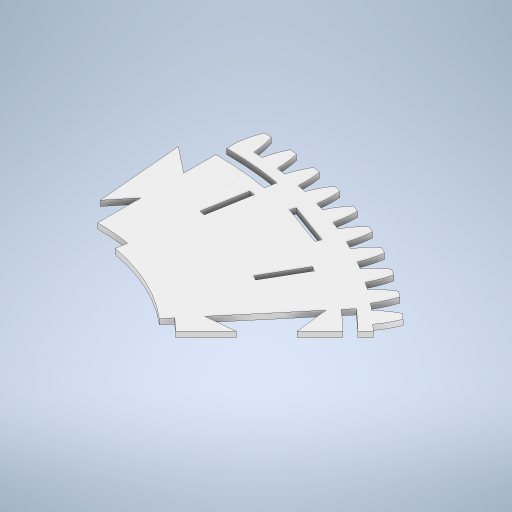
# Autodesk Inventor part: Base Plate Bottom v3
Saved by Autodesk Inventor 2023 (Build 270158000, 158)
## iProperties
Created: 2023-02-13
Part Number: Base Plate Bottom v3
Material: LCP Plastic
Document SubType Name: Sheet Metal
Designer: cheng
Density: 1.626 g/cm^3
Appearance: Smooth - White
Sheet Metal Rule: Default
Author: cheng
Autodesk Inventor part; units mm, degrees
ref_plane "YZ Plane" through (0, 0, 0) normal (1, 0, 0) x (0, 1, 0)
ref_plane "XZ Plane" through (0, 0, 0) normal (0, 1, 0) x (-1, 0, 0)
ref_plane "XY Plane" through (0, 0, 0) normal (0, 0, 1) x (1, 0, 0)
sketch "Sketch2" plane through (0, 0, 0) normal (0, 1, 0) x (-1, 0, 0)
  circle A0 centre (0, 0) radius 325
  circle A1 centre (0, 0) radius 165
  line L0 (0, 0) -> (0, -325)
  line L1 (0, 0) -> (-229.8097, -229.8097)
  line L2 (0, 0) -> (28.3256, -323.7633)
  line L3 (0, 0) -> (-208.906, -248.9644)
  circle A2 centre (0, 0) radius 275 construction
  circle A3 centre (0, 0) radius 195
  circle A4 centre (0, 0) radius 215
  circle A5 centre (0, 0) radius 255 construction
  line L4 (16.9954, -194.258) -> (0, -215)
  line L5 (23.9678, -273.9535) -> (0, -255)
  line L6 (-125.3436, -149.3787) -> (-152.028, -152.028)
  line L7 (-176.7666, -210.6622) -> (-180.3122, -180.3122)
  line L8 (0, 0) -> (-111.1565, -305.4001) construction
  circle A6 centre (0, 0) radius 235 construction
  circle A7 centre (0, 0) radius 275 construction
  line L9 (0, 0) -> (-17.0092, -324.5546) construction
  line L10 (0, 0) -> (-8.5075, -324.8886) construction
  circle A8 centre (0, 0) radius 305
  arc A9 (-5.1732, -324.9588) -> (0, -305) centre (-79.3819, -295.0744) ccw
  arc A10 (-15.9625, -304.582) -> (-11.8409, -324.7842) centre (63.8301, -298.8246) ccw
  arc A11 (20.3387, -324.363) -> (23.93, -304.0598) centre (-55.9859, -300.393) ccw
  arc A12 (7.984, -304.8955) -> (13.6779, -324.712) centre (87.0788, -292.8953) ccw
  arc A13 (45.7252, -321.7673) -> (47.7125, -301.2449) centre (-32.2447, -303.8596) ccw
  arc A14 (31.8812, -303.3292) -> (39.1123, -322.6379) centre (109.7907, -285.1603) ccw
  arc A15 (70.8298, -317.1879) -> (71.2008, -296.5728) centre (-8.3048, -305.4528) ccw
  arc A16 (55.5818, -299.8927) -> (64.3057, -318.5746) centre (131.8257, -275.6672) ccw
  arc A17 (95.4978, -310.6528) -> (94.2502, -290.0722) centre (15.6864, -305.1628) ccw
  arc A18 (78.9398, -294.6074) -> (89.1025, -312.5472) centre (153.0479, -264.4745) ccw
  arc A19 (119.5769, -302.2025) -> (116.7184, -281.7833) centre (39.5808, -302.9913) ccw
  arc A20 (101.8111, -287.5057) -> (113.35, -304.5928) centre (173.3265, -251.6512) ccw
  arc A21 (142.9188, -291.889) -> (138.4671, -271.757) centre (63.2312, -298.9518) ccw
  arc A22 (124.0547, -278.6314) -> (136.8987, -294.7605) centre (192.5365, -237.2764) ccw
  arc A23 (165.3796, -279.776) -> (159.3621, -260.0553) centre (86.4918, -293.0692) ccw
  arc A24 (145.5334, -268.0392) -> (159.6033, -283.1109) centre (210.5595, -221.4387) ccw
  arc A25 (186.8208, -265.938) -> (179.2745, -246.7502) centre (109.2191, -285.3797) ccw
  arc A26 (166.1149, -255.7945) -> (181.3239, -269.7159) centre (227.2843, -204.2358) ccw
  arc A27 (207.1101, -250.4604) -> (198.0817, -231.9238) centre (131.273, -275.9308) ccw
  arc A28 (185.6722, -241.9728) -> (201.9266, -254.6579) centre (242.6078, -185.7736) ccw
  arc A29 (226.1226, -233.4386) -> (215.6676, -215.6676) centre (152.5177, -264.7806) ccw
  arc A30 (204.0848, -226.6592) -> (221.2844, -238.0299) centre (256.4356, -166.1662) ccw
  arc A31 (243.7409, -214.9776) -> (231.9238, -198.0817) centre (172.8219, -251.998) ccw
  arc A32 (221.2392, -209.9481) -> (239.2778, -219.9344) centre (268.6823, -145.5342) ccw
  arc A33 (259.8565, -195.1912) -> (246.7502, -179.2745) centre (192.0607, -237.6617) ccw
  arc A34 (237.0295, -191.9427) -> (255.7961, -200.4829) centre (279.2725, -124.005) ccw
  arc A35 (274.3699, -174.2014) -> (260.0553, -159.3621) centre (210.1154, -221.8601) ccw
  arc A36 (251.3585, -172.7539) -> (270.7372, -179.7953) centre (288.1409, -101.7113) ccw
  arc A37 (287.1918, -152.1376) -> (271.757, -138.4671) centre (226.8746, -204.6908) ccw
  arc A38 (264.1377, -152.5) -> (284.0092, -157.9993) centre (295.2329, -78.7905) ccw
  arc A39 (298.2431, -129.1358) -> (281.7833, -116.7184) centre (242.2351, -186.2594) ccw
  arc A40 (275.2885, -131.3059) -> (295.5302, -135.2291) centre (300.5046, -55.3839) ccw
  arc A41 (307.4556, -105.3378) -> (290.0722, -94.2502) centre (256.1021, -166.6797) ccw
  arc A42 (284.742, -109.3022) -> (305.2291, -111.6252) centre (303.9236, -31.6358) ccw
  arc A43 (314.7725, -80.8904) -> (296.5728, -71.2008) centre (268.3902, -146.0723) ccw
  arc A44 (292.44, -86.6247) -> (313.0462, -87.3331) centre (305.4688, -7.6927) ccw
  arc A45 (320.1488, -55.9443) -> (301.2449, -47.7125) centre (279.0235, -124.5644) ccw
  arc A46 (298.335, -63.4131) -> (318.9333, -62.5025) centre (305.1308, 16.2978) ccw
  arc A47 (323.5512, -30.6533) -> (304.0598, -23.93) centre (287.9366, -102.2884) ccw
  arc A48 (302.3907, -39.8105) -> (322.854, -37.2867) centre (302.9114, 40.1878) ccw
  arc A49 (324.9588, -5.1732) -> (305, 0) centre (295.0744, -79.3819) ccw
  arc A50 (304.582, -15.9625) -> (324.7842, -11.8409) centre (298.8246, 63.8301) ccw
  arc A51 (324.363, 20.3387) -> (304.0598, 23.93) centre (300.393, -55.9859) ccw
  arc A52 (304.8955, 7.984) -> (324.712, 13.6779) centre (292.8953, 87.0788) ccw
  arc A53 (321.7673, 45.7252) -> (301.2449, 47.7125) centre (303.8596, -32.2447) ccw
  arc A54 (303.3292, 31.8812) -> (322.6379, 39.1123) centre (285.1603, 109.7907) ccw
  arc A55 (317.1879, 70.8298) -> (296.5728, 71.2008) centre (305.4528, -8.3048) ccw
  arc A56 (299.8927, 55.5818) -> (318.5746, 64.3057) centre (275.6672, 131.8257) ccw
  arc A57 (310.6528, 95.4978) -> (290.0722, 94.2502) centre (305.1628, 15.6864) ccw
  arc A58 (294.6074, 78.9398) -> (312.5472, 89.1025) centre (264.4745, 153.0479) ccw
  arc A59 (302.2025, 119.5769) -> (281.7833, 116.7184) centre (302.9913, 39.5808) ccw
  arc A60 (287.5057, 101.8111) -> (304.5928, 113.35) centre (251.6512, 173.3265) ccw
  arc A61 (291.889, 142.9188) -> (271.757, 138.4671) centre (298.9518, 63.2312) ccw
  arc A62 (278.6314, 124.0547) -> (294.7605, 136.8987) centre (237.2764, 192.5365) ccw
  arc A63 (279.776, 165.3796) -> (260.0553, 159.3621) centre (293.0692, 86.4918) ccw
  arc A64 (268.0392, 145.5334) -> (283.1109, 159.6033) centre (221.4387, 210.5595) ccw
  arc A65 (265.938, 186.8208) -> (246.7502, 179.2745) centre (285.3797, 109.2191) ccw
  arc A66 (255.7945, 166.1149) -> (269.7159, 181.3239) centre (204.2358, 227.2843) ccw
  arc A67 (250.4604, 207.1101) -> (231.9238, 198.0817) centre (275.9308, 131.273) ccw
  arc A68 (241.9728, 185.6722) -> (254.6579, 201.9266) centre (185.7736, 242.6078) ccw
  arc A69 (233.4386, 226.1226) -> (215.6676, 215.6676) centre (264.7806, 152.5177) ccw
  arc A70 (226.6592, 204.0848) -> (238.0299, 221.2844) centre (166.1662, 256.4356) ccw
  arc A71 (214.9776, 243.7409) -> (198.0817, 231.9238) centre (251.998, 172.8219) ccw
  arc A72 (209.9481, 221.2392) -> (219.9344, 239.2778) centre (145.5342, 268.6823) ccw
  arc A73 (195.1912, 259.8565) -> (179.2745, 246.7502) centre (237.6617, 192.0607) ccw
  arc A74 (191.9427, 237.0295) -> (200.4829, 255.7961) centre (124.005, 279.2725) ccw
  arc A75 (174.2014, 274.3699) -> (159.3621, 260.0553) centre (221.8601, 210.1154) ccw
  arc A76 (172.7539, 251.3585) -> (179.7953, 270.7372) centre (101.7113, 288.1409) ccw
  arc A77 (152.1376, 287.1918) -> (138.4671, 271.757) centre (204.6908, 226.8746) ccw
  arc A78 (152.5, 264.1377) -> (157.9993, 284.0092) centre (78.7905, 295.2329) ccw
  arc A79 (129.1358, 298.2431) -> (116.7184, 281.7833) centre (186.2594, 242.2351) ccw
  arc A80 (131.3059, 275.2885) -> (135.2291, 295.5302) centre (55.3839, 300.5046) ccw
  arc A81 (105.3378, 307.4556) -> (94.2502, 290.0722) centre (166.6797, 256.1021) ccw
  arc A82 (109.3022, 284.742) -> (111.6252, 305.2291) centre (31.6358, 303.9236) ccw
  arc A83 (80.8904, 314.7725) -> (71.2008, 296.5728) centre (146.0723, 268.3902) ccw
  arc A84 (86.6247, 292.44) -> (87.3331, 313.0462) centre (7.6927, 305.4688) ccw
  arc A85 (55.9443, 320.1488) -> (47.7125, 301.2449) centre (124.5644, 279.0235) ccw
  arc A86 (63.4131, 298.335) -> (62.5025, 318.9333) centre (-16.2978, 305.1308) ccw
  arc A87 (30.6533, 323.5512) -> (23.93, 304.0598) centre (102.2884, 287.9366) ccw
  arc A88 (39.8105, 302.3907) -> (37.2867, 322.854) centre (-40.1878, 302.9114) ccw
  circle A89 centre (0, 0) radius 295
  circle A90 centre (0, 0) radius 285
  line L11 (0, 0) -> (-52.9627, -300.3664)
  line L12 (-80.392, -279.3513) -> (-117.9797, -265.6705)
  line L13 (-117.9797, -265.6705) -> (-116.2696, -260.972)
  line L14 (-116.2696, -260.972) -> (-78.6819, -274.6528)
  line L15 (-78.6819, -274.6528) -> (-80.392, -279.3513)
  line L16 (-80.392, -279.3513) -> (-116.2696, -260.972) construction
  line L17 (-117.9797, -265.6705) -> (-78.6819, -274.6528) construction
  line L18 (-98.3308, -270.1616) -> (-99.1858, -272.5109)
  circle A91 centre (0, 0) radius 175
  line L19 (-135.3349, -239.407) -> (-139.6651, -236.907)
  line L20 (-139.6651, -236.907) -> (-119.6651, -202.266)
  line L21 (-119.6651, -202.266) -> (-115.3349, -204.766)
  line L22 (-115.3349, -204.766) -> (-135.3349, -239.407)
  line L23 (-135.3349, -239.407) -> (-119.6651, -202.266) construction
  line L24 (-139.6651, -236.907) -> (-115.3349, -204.766) construction
  line L25 (-137.5, -238.157) -> (-117.5, -203.516) construction
  line L26 (-129.6651, -219.5865) -> (-125.3349, -222.0865) construction
  line L27 (-50.2153, -270.388) -> (-45.2912, -271.2563)
  line L28 (-45.2912, -271.2563) -> (-38.3453, -231.8639)
  line L29 (-38.3453, -231.8639) -> (-43.2693, -230.9957)
  line L30 (-43.2693, -230.9957) -> (-50.2153, -270.388)
  line L31 (-50.2153, -270.388) -> (-38.3453, -231.8639) construction
  line L32 (-45.2912, -271.2563) -> (-43.2693, -230.9957) construction
  line L33 (-47.7532, -270.8221) -> (-40.8073, -231.4298) construction
  arc A92 (5.1732, 324.9588) -> (0, 305) centre (79.3819, 295.0744) ccw
  arc A93 (15.9625, 304.582) -> (11.8409, 324.7842) centre (-63.8301, 298.8246) ccw
  arc A94 (-20.3387, 324.363) -> (-23.93, 304.0598) centre (55.9859, 300.393) ccw
  arc A95 (-7.984, 304.8955) -> (-13.6779, 324.712) centre (-87.0788, 292.8953) ccw
  arc A96 (-45.7252, 321.7673) -> (-47.7125, 301.2449) centre (32.2447, 303.8596) ccw
  arc A97 (-31.8812, 303.3292) -> (-39.1123, 322.6379) centre (-109.7907, 285.1603) ccw
  arc A98 (-70.8298, 317.1879) -> (-71.2008, 296.5728) centre (8.3048, 305.4528) ccw
  arc A99 (-55.5818, 299.8927) -> (-64.3057, 318.5746) centre (-131.8257, 275.6672) ccw
  arc A100 (-95.4978, 310.6528) -> (-94.2502, 290.0722) centre (-15.6864, 305.1628) ccw
  arc A101 (-78.9398, 294.6074) -> (-89.1025, 312.5472) centre (-153.0479, 264.4745) ccw
  arc A102 (-119.5769, 302.2025) -> (-116.7184, 281.7833) centre (-39.5808, 302.9913) ccw
  arc A103 (-101.8111, 287.5057) -> (-113.35, 304.5928) centre (-173.3265, 251.6512) ccw
  arc A104 (-142.9188, 291.889) -> (-138.4671, 271.757) centre (-63.2312, 298.9518) ccw
  arc A105 (-124.0547, 278.6314) -> (-136.8987, 294.7605) centre (-192.5365, 237.2764) ccw
  arc A106 (-165.3796, 279.776) -> (-159.3621, 260.0553) centre (-86.4918, 293.0692) ccw
  arc A107 (-145.5334, 268.0392) -> (-159.6033, 283.1109) centre (-210.5595, 221.4387) ccw
  arc A108 (-186.8208, 265.938) -> (-179.2745, 246.7502) centre (-109.2191, 285.3797) ccw
  arc A109 (-166.1149, 255.7945) -> (-181.3239, 269.7159) centre (-227.2843, 204.2358) ccw
  arc A110 (-207.1101, 250.4604) -> (-198.0817, 231.9238) centre (-131.273, 275.9308) ccw
  arc A111 (-185.6722, 241.9728) -> (-201.9266, 254.6579) centre (-242.6078, 185.7736) ccw
  arc A112 (-226.1226, 233.4386) -> (-215.6676, 215.6676) centre (-152.5177, 264.7806) ccw
  arc A113 (-204.0848, 226.6592) -> (-221.2844, 238.0299) centre (-256.4356, 166.1662) ccw
  arc A114 (-243.7409, 214.9776) -> (-231.9238, 198.0817) centre (-172.8219, 251.998) ccw
  arc A115 (-221.2392, 209.9481) -> (-239.2778, 219.9344) centre (-268.6823, 145.5342) ccw
  arc A116 (-259.8565, 195.1912) -> (-246.7502, 179.2745) centre (-192.0607, 237.6617) ccw
  arc A117 (-237.0295, 191.9427) -> (-255.7961, 200.4829) centre (-279.2725, 124.005) ccw
  arc A118 (-274.3699, 174.2014) -> (-260.0553, 159.3621) centre (-210.1154, 221.8601) ccw
  arc A119 (-251.3585, 172.7539) -> (-270.7372, 179.7953) centre (-288.1409, 101.7113) ccw
  arc A120 (-287.1918, 152.1376) -> (-271.757, 138.4671) centre (-226.8746, 204.6908) ccw
  arc A121 (-264.1377, 152.5) -> (-284.0092, 157.9993) centre (-295.2329, 78.7905) ccw
  arc A122 (-298.2431, 129.1358) -> (-281.7833, 116.7184) centre (-242.2351, 186.2594) ccw
  arc A123 (-275.2885, 131.3059) -> (-295.5302, 135.2291) centre (-300.5046, 55.3839) ccw
  arc A124 (-307.4556, 105.3378) -> (-290.0722, 94.2502) centre (-256.1021, 166.6797) ccw
  arc A125 (-284.742, 109.3022) -> (-305.2291, 111.6252) centre (-303.9236, 31.6358) ccw
  arc A126 (-314.7725, 80.8904) -> (-296.5728, 71.2008) centre (-268.3902, 146.0723) ccw
  arc A127 (-292.44, 86.6247) -> (-313.0462, 87.3331) centre (-305.4688, 7.6927) ccw
  arc A128 (-320.1488, 55.9443) -> (-301.2449, 47.7125) centre (-279.0235, 124.5644) ccw
  arc A129 (-298.335, 63.4131) -> (-318.9333, 62.5025) centre (-305.1308, -16.2978) ccw
  arc A130 (-323.5512, 30.6533) -> (-304.0598, 23.93) centre (-287.9366, 102.2884) ccw
  arc A131 (-302.3907, 39.8105) -> (-322.854, 37.2867) centre (-302.9114, -40.1878) ccw
  arc A132 (-324.9588, 5.1732) -> (-305, 0) centre (-295.0744, 79.3819) ccw
  arc A133 (-304.582, 15.9625) -> (-324.7842, 11.8409) centre (-298.8246, -63.8301) ccw
  arc A134 (-324.363, -20.3387) -> (-304.0598, -23.93) centre (-300.393, 55.9859) ccw
  arc A135 (-304.8955, -7.984) -> (-324.712, -13.6779) centre (-292.8953, -87.0788) ccw
  arc A136 (-321.7673, -45.7252) -> (-301.2449, -47.7125) centre (-303.8596, 32.2447) ccw
  arc A137 (-303.3292, -31.8812) -> (-322.6379, -39.1123) centre (-285.1603, -109.7907) ccw
  arc A138 (-317.1879, -70.8298) -> (-296.5728, -71.2008) centre (-305.4528, 8.3048) ccw
  arc A139 (-299.8927, -55.5818) -> (-318.5746, -64.3057) centre (-275.6672, -131.8257) ccw
  arc A140 (-310.6528, -95.4978) -> (-290.0722, -94.2502) centre (-305.1628, -15.6864) ccw
  arc A141 (-294.6074, -78.9398) -> (-312.5472, -89.1025) centre (-264.4745, -153.0479) ccw
  arc A142 (-302.2025, -119.5769) -> (-281.7833, -116.7184) centre (-302.9913, -39.5808) ccw
  arc A143 (-287.5057, -101.8111) -> (-304.5928, -113.35) centre (-251.6512, -173.3265) ccw
  arc A144 (-291.889, -142.9188) -> (-271.757, -138.4671) centre (-298.9518, -63.2312) ccw
  arc A145 (-278.6314, -124.0547) -> (-294.7605, -136.8987) centre (-237.2764, -192.5365) ccw
  arc A146 (-279.776, -165.3796) -> (-260.0553, -159.3621) centre (-293.0692, -86.4918) ccw
  arc A147 (-268.0392, -145.5334) -> (-283.1109, -159.6033) centre (-221.4387, -210.5595) ccw
  arc A148 (-265.938, -186.8208) -> (-246.7502, -179.2745) centre (-285.3797, -109.2191) ccw
  arc A149 (-255.7945, -166.1149) -> (-269.7159, -181.3239) centre (-204.2358, -227.2843) ccw
  arc A150 (-250.4604, -207.1101) -> (-231.9238, -198.0817) centre (-275.9308, -131.273) ccw
  arc A151 (-241.9728, -185.6722) -> (-254.6579, -201.9266) centre (-185.7736, -242.6078) ccw
  arc A152 (-233.4386, -226.1226) -> (-215.6676, -215.6676) centre (-264.7806, -152.5177) ccw
  arc A153 (-226.6592, -204.0848) -> (-238.0299, -221.2844) centre (-166.1662, -256.4356) ccw
  arc A154 (-214.9776, -243.7409) -> (-198.0817, -231.9238) centre (-251.998, -172.8219) ccw
  arc A155 (-209.9481, -221.2392) -> (-219.9344, -239.2778) centre (-145.5342, -268.6823) ccw
  arc A156 (-195.1912, -259.8565) -> (-179.2745, -246.7502) centre (-237.6617, -192.0607) ccw
  arc A157 (-191.9427, -237.0295) -> (-200.4829, -255.7961) centre (-124.005, -279.2725) ccw
  arc A158 (-174.2014, -274.3699) -> (-159.3621, -260.0553) centre (-221.8601, -210.1154) ccw
  arc A159 (-172.7539, -251.3585) -> (-179.7953, -270.7372) centre (-101.7113, -288.1409) ccw
  arc A160 (-152.1376, -287.1918) -> (-138.4671, -271.757) centre (-204.6908, -226.8746) ccw
  arc A161 (-152.5, -264.1377) -> (-157.9993, -284.0092) centre (-78.7905, -295.2329) ccw
  arc A162 (-129.1358, -298.2431) -> (-116.7184, -281.7833) centre (-186.2594, -242.2351) ccw
  arc A163 (-131.3059, -275.2885) -> (-135.2291, -295.5302) centre (-55.3839, -300.5046) ccw
  arc A164 (-105.3378, -307.4556) -> (-94.2502, -290.0722) centre (-166.6797, -256.1021) ccw
  arc A165 (-109.3022, -284.742) -> (-111.6252, -305.2291) centre (-31.6358, -303.9236) ccw
  arc A166 (-80.8904, -314.7725) -> (-71.2008, -296.5728) centre (-146.0723, -268.3902) ccw
  arc A167 (-86.6247, -292.44) -> (-87.3331, -313.0462) centre (-7.6927, -305.4688) ccw
  arc A168 (-55.9443, -320.1488) -> (-47.7125, -301.2449) centre (-124.5644, -279.0235) ccw
  arc A169 (-63.4131, -298.335) -> (-62.5025, -318.9333) centre (16.2978, -305.1308) ccw
  arc A170 (-30.6533, -323.5512) -> (-23.93, -304.0598) centre (-102.2884, -287.9366) ccw
  arc A171 (-39.8105, -302.3907) -> (-37.2867, -322.854) centre (40.1878, -302.9114) ccw
  point P0 (0, -165)
  point P1 (-116.6726, -116.6726)
  point P2 (-215.6676, -215.6676)
  point P3 (109.3022, 284.742)
  point P4 (111.6252, 305.2291)
  point P5 (105.3378, 307.4556)
  point P6 (94.2502, 290.0722)
  point P7 (86.6247, 292.44)
  point P8 (87.3331, 313.0462)
  point P9 (80.8904, 314.7725)
  point P10 (71.2008, 296.5728)
  point P11 (63.4131, 298.335)
  point P12 (62.5025, 318.9333)
  point P13 (55.9443, 320.1488)
  point P14 (47.7125, 301.2449)
  point P15 (39.8105, 302.3907)
  point P16 (37.2867, 322.854)
  point P17 (30.6533, 323.5512)
  point P18 (23.93, 304.0598)
  point P19 (-15.9625, -304.582)
  point P20 (-11.8409, -324.7842)
  point P21 (-37.3344, -211.7337)
  point P22 (-201.5254, -201.5254)
  point P23 (-183.1945, -218.3227)
  point P24 (-189.6223, -225.9831)
  point P25 (-208.5965, -208.5965)
  point P26 (0, -295)
  point P27 (-51.2262, -290.5183)
  point P28 (-49.4897, -280.6702)
  point P29 (0, -285)
  point P30 (0, -175)
  point P31 (-30.3884, -172.3414)
  point P32 (-28.6519, -162.4933)
  point P33 (-106.06, -126.3973)
  point P34 (-112.4878, -134.0578)
  point P35 (-123.7437, -123.7437)
  point P36 (-127.5, -220.8365)
  point P37 (15.2523, -174.3341)
  point P38 (-196.0502, -233.6436)
  point P39 (26.5825, -303.8394)
  point P40 (25.7109, -293.8774)
  point P41 (24.8394, -283.9155)
  point P42 (14.3807, -164.3721)
  point P43 (-219.9344, -239.2778)
  point P44 (-198.0817, -231.9238)
  point P45 (-200.4829, -255.7961)
  point P46 (-195.1912, -259.8565)
  point P47 (-179.2745, -246.7502)
  point P48 (-172.7539, -251.3585)
  point P49 (-179.7953, -270.7372)
  point P50 (-174.2014, -274.3699)
  point P51 (-152.5, -264.1377)
  point P52 (-157.9993, -284.0092)
  point P53 (-138.4671, -271.757)
  point P54 (-135.2291, -295.5302)
  point P55 (-116.7184, -281.7833)
  point P56 (-109.3022, -284.742)
  point P57 (-111.6252, -305.2291)
  point P58 (-105.3378, -307.4556)
  point P59 (-94.2502, -290.0722)
  point P60 (-86.6247, -292.44)
  point P61 (-87.3331, -313.0462)
  point P62 (-80.8904, -314.7725)
  point P63 (-71.2008, -296.5728)
  point P64 (-63.4131, -298.335)
  point P65 (-62.5025, -318.9333)
  point P66 (-55.9443, -320.1488)
  point P67 (-47.7125, -301.2449)
  point P68 (-37.2867, -322.854)
  point P69 (-23.93, -304.0598)
  dimension "d0" = 650
  dimension "d42" = 20
  dimension "d57" = 90
  dimension "d1" = 330
  dimension "d2" = 45
  dimension "d3" = 5
  dimension "d4" = 5
  dimension "d6" = 30
  dimension "d7" = 20
  dimension "d8" = 20
  dimension "d14" = 20
  dimension "d35" = 3
  dimension "d36" = 1.5
  dimension "d44" = 80
  dimension "d47" = 360
  dimension "d50" = 10
  dimension "d52" = 10
  dimension "d53" = 40
  dimension "d54" = 5
  dimension "d55" = 10
  dimension "d61" = 40
  dimension "d63" = 5
  dimension "d64" = 10
  dimension "d66" = 40
  constraints: 329 point on circle, 169 centre point, 68 end point, 13 coincident, 9 midpoint, 9 point on line, 9 symmetric about line, 4 parallel, 2 perpendicular, 2 tangent, 1 collinear, 1 vertical, 659 other
  measures "d1" diameter of A1
  measures "d2" angle of L1 L0
  measures "d3" angle of L2 L0
  measures "d4" angle of L1 L3
  measures "d6" radial gap between concentric circles of A3 A1
  measures "d7" radial gap between concentric circles of A3 A4
  measures "d8" radial gap between concentric circles of A5 A2
  measures "d14" angle of L3 L8
  measures "d35" angle of L0 L9
  measures "d36" angle of L9 L10
  measures "d44" radius of A9
  measures "d50" radial gap between concentric circles of A90 A89
  measures "d52" angle of L11 L0
  measures "d53" distance of L12.start L12.end
  measures "d54" distance between parallel lines of L12 L14
  measures "d55" radial gap between concentric circles of A91 A1
  measures "d63" distance between parallel lines of L22 L20
  measures "d64" angle of L22 L8
extrude "Extrusion1" add sketch "Sketch2" along normal blind 5 contours L0 A8 L11 A89 | A0 A10 A8 A9 | L5 L0 A4 L2 | A90 L11 L27 L28 L29 A4 L0 | L11 A8 L3 A89 | A89 L3 A90 L11 | A89 L3 A8 L1 | A4 L4 L2 | A90 L3 A4 L11 L29 L30 L27 | L1 L7 L3 A90 | A8 A168 A0 A169 | A0 A171 A8 A170 | A4 L11 A3 L0 | A8 A154 A0 A155 | A3 L11 A91 L0 | A4 L3 A3 L11 | L1 A3 L6 | A8 A156 A0 A157 | A166 A0 A167 A8 | L1 A91 L3 A3 | A3 L3 A91 L11 | A91 L3 A1 L11 | A8 A158 A0 A159 | A164 A0 A165 A8 | A8 A160 A0 A161 | A162 A0 A163 A8
body "Solid1"
